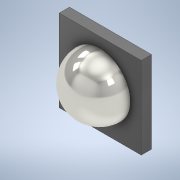
# Autodesk Inventor part: button 2
Saved by Autodesk Inventor 2021 (Build 250183000, 183)
## iProperties
Created: 2021-07-11
Part Number: button 2
Material: Generic
Document SubType Name: Modeling
Designer: Manojgouda K R
Density: 1 g/cm^3
Appearance: Default
Author: Manojgouda K R
Autodesk Inventor part; units mm, degrees
ref_plane "YZ Plane" through (0, 0, 0) normal (1, 0, 0) x (0, 1, 0)
ref_plane "XZ Plane" through (0, 0, 0) normal (0, 1, 0) x (-1, 0, 0)
ref_plane "XY Plane" through (0, 0, 0) normal (0, 0, 1) x (1, 0, 0)
sketch "Sketch1" plane through (0, 0, 0) normal (0, 0, 1) x (1, 0, 0)
  line L0 (-3.4074, 2.2935) -> (-1.4074, 2.2935)
  line L1 (-1.4074, 2.2935) -> (-1.4074, 0.2935)
  line L2 (-1.4074, 0.2935) -> (-3.4074, 0.2935)
  line L3 (-3.4074, 0.2935) -> (-3.4074, 2.2935)
  point P0 (0, 0)
  dimension "d0" = 2
  dimension "d1" = 2
  constraints: 8 end point, 2 parallel, 1 horizontal, 1 perpendicular
  measures "d0" distance of L1.end L2.end
  measures "d1" distance of L0.end L1.end
extrude "Extrusion1" add sketch "Sketch1" along normal blind 0.25
sketch "Sketch2" plane through (0, 0, 0.25) normal (0, 0, 1) x (1, 0, 0)
  arc A0 (-2.4236, 0.5435) -> (-2.4236, 2.0435) centre (-2.4236, 1.2935) ccw
  line L0 (-2.4236, 2.0435) -> (-2.4236, 0.5435)
  point P0 (0, 0)
  dimension "d5" = 1.5
  constraints: 2 end point, 2 point on circle, 1 centre point, 1 vertical
  measures "d5" diameter of A0
revolve "Revolution1" add sketch "Sketch2" angle 180 about axis through (-2.4236, 2.0435, 0.25) along (0, -1, 0)
body "Solid1"
